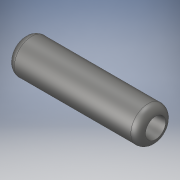
# Autodesk Inventor part: handle bar
Saved by Autodesk Inventor 2017 (Build 210142000, 142)
## iProperties
Created: 2017-01-09
Part Number: handle bar
Material: Rubber
Document SubType Name: Modeling
Designer: 193515
Density: 0.93 g/cm^3
Appearance: Rubber - Black - Version 1.1
Author: 193515
Autodesk Inventor part; units mm, degrees
ref_plane "YZ Plane" through (0, 0, 0) normal (1, 0, 0) x (0, 1, 0)
ref_plane "XZ Plane" through (0, 0, 0) normal (0, 1, 0) x (-1, 0, 0)
ref_plane "XY Plane" through (0, 0, 0) normal (0, 0, 1) x (1, 0, 0)
sketch "Sketch1" plane through (0, 0, 0) normal (0, 0, 1) x (1, 0, 0)
  line L0 (-3.5739, 7.4603) -> (-3.5739, -5.2397)
  line L1 (-3.5739, -5.2397) -> (109.9387, -5.2397)
  line L2 (109.9387, -5.2397) -> (109.9387, 1.1103)
  line L3 (109.9387, 1.1103) -> (0.3885, 1.1103)
  line L4 (0.3885, 1.1103) -> (0.3885, 7.4603)
  line L5 (0.3885, 7.4603) -> (-3.5739, 7.4603)
  line L6 (-3.5739, 7.4603) -> (-3.5739, 9.8416)
  line L7 (-3.5739, 9.8416) -> (113.4449, 9.8416)
  point P0 (0, 0)
  dimension "d0" = 3.9624
  dimension "d1" = 113.5126
  dimension "d2" = 6.35
  dimension "d3" = 12.7
  dimension "d4" = 2.3813
  constraints: 16 end point, 6 perpendicular, 2 vertical
  measures "d0" distance between parallel lines of L4 L0
  measures "d1" distance between parallel lines of L2 L0
  measures "d2" distance between parallel lines of L1 L3
  measures "d3" distance of L0.end L0.start
  measures "d4" distance of L0.start L6.end
revolve "Revolution1" add sketch "Sketch1" angle 360 about axis through (-3.5739, 9.8416, 0) along (1, 0, 0)
fillet "Fillet1" radius 6.35 1 edges at (109.9387, 24.9228, 0)
fillet "Fillet2" radius 6.35 1 edges at (-3.5739, 24.9228, 0)
body "Solid1"
